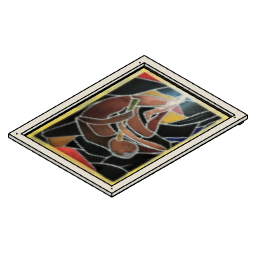
Fluist (Autodesk Fusion 360 archive; units mm, degrees)
design "FensterRekonstruktion"
Autodesk Fusion 360 part; units mm, degrees
sketch "Sketch1" plane through (0, 0, 0) normal (0, 1, 0) x (1, 0, 0)
  line L0 (0, 0) -> (981, 0)
  line L1 (981, 0) -> (981, 1289)
  line L2 (981, 1289) -> (0, 1289)
  line L3 (0, 1289) -> (0, 0)
  line L4 (60, 60) -> (921, 60)
  line L5 (921, 60) -> (921, 1229)
  line L6 (921, 1229) -> (60, 1229)
  line L7 (60, 1229) -> (60, 60)
  line L8 (910.5, 1214.5) -> (70.5, 1214.5)
  line L9 (70.5, 1214.5) -> (70.5, 74.5)
  line L10 (70.5, 74.5) -> (910.5, 74.5)
  line L11 (910.5, 74.5) -> (910.5, 1214.5)
  line L12 (963.5, 1269.5) -> (17.5, 1269.5)
  line L13 (17.5, 1269.5) -> (17.5, 19.5)
  line L14 (17.5, 19.5) -> (963.5, 19.5)
  line L15 (963.5, 19.5) -> (963.5, 1269.5)
  line L16 (17.5, 1269.5) -> (963.5, 1269.5)
  line L17 (963.5, 1269.5) -> (963.5, 20.8056)
  line L18 (963.5, 20.8056) -> (17.5, 20.8056)
  line L19 (17.5, 20.8056) -> (17.5, 1269.5)
  line L20 (981, 1289) -> (490.5, 1289)
  line L21 (490.5, 1289) -> (490.5, 644.5)
  line L22 (490.5, 644.5) -> (981, 644.5)
  line L23 (981, 644.5) -> (981, 1289)
  circle A0 centre (941, 1209) radius 4
  circle A1 centre (941, 40) radius 4
  circle A2 centre (40, 1209) radius 4
  circle A3 centre (40, 40) radius 4
  line L24 (963.5, 1269.5) -> (17.5, 1269.5)
  line L25 (17.5, 1269.5) -> (17.5, 1229.5)
  line L26 (17.5, 1229.5) -> (963.5, 1229.5)
  line L27 (963.5, 1229.5) -> (963.5, 1269.5)
  point P0 (40, 1209)
  point P1 (40, 40)
  dimension "d1" = 1289
  dimension "d2" = 981
  dimension "d3" = 60
  dimension "d4" = 60
  dimension "d5" = 60
  dimension "d6" = 60
  dimension "d14" = 1140
  dimension "d15" = 840
  dimension "d16" = 70.5
  dimension "d17" = 74.5
  dimension "d18" = 1250
  dimension "d19" = 946
  dimension "d20" = 17.5
  dimension "d21" = 19.5
  dimension "d30" = 490.5
  dimension "d31" = 644.5
  dimension "d32" = 8
  dimension "d33" = 80
  dimension "d34" = 40
  dimension "d35" = 8
  dimension "d36" = 40
  dimension "d37" = 40
  dimension "d38" = 8
  dimension "d39" = 8
  dimension "d44" = 40
  constraint horizontal L0
  constraint vertical L1
  constraint horizontal L2
  constraint vertical L3
  constraint coincident L0.start L3.end
  constraint horizontal L4
  constraint vertical L5
  constraint horizontal L6
  constraint vertical L7
  constraint horizontal L8
  constraint vertical L9
  constraint horizontal L10
  constraint vertical L11
  constraint horizontal L12
  constraint vertical L13
  constraint horizontal L14
  constraint vertical L15
  constraint horizontal L16
  constraint vertical L17
  constraint horizontal L18
  constraint vertical L19
  constraint coincident L15 L17.end
  constraint horizontal L20
  constraint vertical L21
  constraint horizontal L22
  constraint vertical L23
  constraint symmetric L21 A0.centre P0
  constraint symmetric L21 A1.centre P1
  constraint coincident P0 A2.centre
  constraint coincident P1 A3.centre
  constraint horizontal L24
  constraint vertical L25
  constraint horizontal L26
  constraint vertical L27
  constraint coincident L19 L25.end
  measures "d1" distance of L0.end L1.end
  measures "d2" distance of L1.end L2.end
  measures "d3" distance of L0 L4
  measures "d4" distance of L3 L7
  measures "d5" distance of L2 L6
  measures "d6" distance of L1 L5
  measures "d14" distance of L8.end L9.end
  measures "d15" distance of L8.start L8.end
  measures "d16" distance of L1 L11
  measures "d17" distance of L0 L10
  measures "d18" distance of L12.start L14.end
  measures "d19" distance of L12.start L12.end
  measures "d20" distance of L1 L15
  measures "d21" distance of L2 L12
  measures "d30" distance of L21.end L22.end
  measures "d31" distance of L2 L22
  measures "d32" diameter of A0
  measures "d33" distance of L20 A0.centre
  measures "d34" distance of L23 A0.centre
  measures "d35" diameter of A1
  measures "d36" distance of L0 A1.centre
  measures "d37" distance of L1 A1.centre
  measures "d38" diameter of A2
  measures "d39" diameter of A3
  measures "d44" distance of L12 L26
extrude "Extrude1" add sketch "Sketch1" along normal blind 30 contours L0 L1 L2 L3 L12 L13 L14 L15 L16 L17 L19 L21 L22 L24 L25 | L1 L2 L12 L15 L16 L17 L20 L21 L22 L23 L24 L27 | L5 L6 L15 L17 L21 L22 L26 | L4 L5 L6 L7 L13 L15 L17 L18 L19 L21 L22 L26 | L12 L13 L16 L19 L21 L24 L25 L26 | L12 L15 L16 L17 L21 L24 L26 L27 | L13 L14 L15 L18 | A0 | A1 | A2 | A3 makes body 1
extrude "Extrude3" add sketch "Sketch1" against normal blind 20 separate body contours L5 L6 L15 L17 L21 L22 L26 | L4 L5 L6 L7 L13 L15 L17 L18 L19 L21 L22 L26 | L12 L13 L16 L19 L21 L24 L25 L26 | L12 L15 L16 L17 L21 L24 L26 L27 | L13 L14 L15 L18 | A0 | A1 | A2 | A3 makes body 2
extrude "Extrude5" add sketch "Sketch1" along normal blind 5 separate body contours L8 L11 L21 L22 | L8 L9 L10 L11 L21 L22 makes body 3
extrude "Extrude6" add sketch "Sketch1" along normal mid plane 10 separate body contours L5 L6 L8 L11 L21 L22 | L4 L5 L6 L7 L8 L9 L10 L11 L21 L22 makes body 4
extrude "Extrude7" cut sketch "Sketch1" against normal blind 50 contours L5 L6 L8 L11 L21 L22 | L4 L5 L6 L7 L8 L9 L10 L11 L21 L22 | L8 L11 L21 L22 | L8 L9 L10 L11 L21 L22 bodies 2
extrude "Extrude8" cut sketch "Sketch1" along normal mid plane 100 contours A0 | A1 | A2 | A3 bodies 1 2
extrude "Extrude9" add sketch "Sketch1" against normal blind 30 contours L12 L13 L16 L19 L21 L24 L25 L26 | L12 L15 L16 L17 L21 L24 L26 L27 bodies 2
equation "d4 = d3"
equation "d5 = d3"
equation "d6 = d3"
equation "d16 = ( d2 - d15 ) / 2"
equation "d17 = ( d1 - d14 ) / 2"
equation "d20 = ( d2 - d19 ) / 2"
equation "d21 = ( d1 - d18 ) / 2"
equation "d30 = d2 / 2"
equation "d31 = d1 / 2"
named bodies: "Front-Frame", "Back-Frame", "Glas", "GlasFrame"

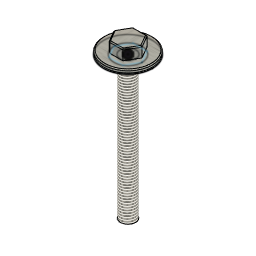
design "Screws"
Autodesk Fusion 360 part; units mm, degrees
sketch "Sketch1" plane through (0, 0, 0) normal (0, 1, 0) x (1, 0, 0)
  circle A0 centre (0, 0) radius 7.19
  line L0 (7.19, 0) -> (3.595, 6.2267)
  line L1 (3.595, 6.2267) -> (-3.595, 6.2267)
  line L2 (-3.595, 6.2267) -> (-7.19, 0)
  line L3 (-7.19, 0) -> (-3.595, -6.2267)
  line L4 (-3.595, -6.2267) -> (3.595, -6.2267)
  line L5 (3.595, -6.2267) -> (7.19, 0)
  circle A1 centre (0, 0) radius 4
  circle A2 centre (0, 0) radius 12.5
  dimension "d1" = 14.38
  dimension "d2" = 8
  dimension "d13" = 25
  constraint coincident A0.centre A1.centre
  constraint coincident A0 L0.start
  constraint concentric A1 A2
  measures "d1" diameter of A0
  measures "d2" diameter of A1
  measures "d13" diameter of A2
extrude "Extrude1" add sketch "Sketch1" along normal blind 5.3 contours L0 L1 L2 L3 L4 L5 | A1 makes body 1
chamfer "Chamfer1" distance 0.5 angle 45 1 edges at (-5.3925, 5.3, 3.1134) 2 faces at (-2.3967, 5.3, 0) (-5.9917, 1.7667, 2.0756) on bodies 1
extrude "Extrude2" add sketch "Sketch1" against normal blind 75 contours A1 bodies 1
thread "Thread1" "ISO Metric profile 8.0 M8x1.25 6g" major diameter 7.866 minor diameter 6.4455 pitch 1.25 angle 60 resizes the face on face at (3.995, -50, 0.1994) on bodies 1
move_body "Move1" bodies 1 to x (1, 0, 0) y (0, 1, 0) z (0, 0, 1) at (0, 2, 0)
extrude "Extrude3" add sketch "Sketch1" along normal blind 2 separate body contours A0 L0 | L0 L1 L2 L3 L4 L5 | A0 L5 | A0 L1 | A0 L4 | A0 L2 | A0 L3 | A2 makes body 2
fillet "Fillet1" radius 0.5 2 edges at (-11.6541, 2, 4.5202) (-11.6541, 0, 4.5202) on bodies 2
move_face "OffsetFaces1" offset -1 1 faces at (3.995, 1.3333, 0.1994) on bodies 2
